Autodesk Inventor part; units mm, degrees
(part 3 of 4)
  line L749 (-36.8358, 2.1011) -> (-36.8212, 2.0626) construction
  line L750 (-36.8212, 2.0626) -> (-36.7965, 1.9968) construction
  line L751 (-36.7965, 1.9968) -> (-36.752, 1.9602) construction
  line L752 (-36.752, 1.9602) -> (-36.6802, 1.9558) construction
  line L753 (-36.6802, 1.9558) -> (-36.5155, 1.9456) construction
  line L754 (-36.5155, 1.9456) -> (-36.351, 1.9258) construction
  line L755 (-36.351, 1.9258) -> (-36.1863, 1.9252) construction
  line L756 (-36.1863, 1.9252) -> (-36.0465, 1.9246) construction
  line L757 (-36.0465, 1.9246) -> (-35.9064, 1.9438) construction
  line L758 (-35.9064, 1.9438) -> (-35.767, 1.9589) construction
  line L759 (-35.767, 1.9589) -> (-35.7495, 1.9609) construction
  line L760 (-35.7495, 1.9609) -> (-35.7233, 1.9899) construction
  line L761 (-35.7233, 1.9899) -> (-35.7209, 2.009) construction
  line L762 (-35.7209, 2.009) -> (-35.7008, 2.1678) construction
  line L763 (-35.7008, 2.1678) -> (-35.7931, 2.3069) construction
  line L764 (-35.7931, 2.3069) -> (-35.9501, 2.3398) construction
  line L765 (-35.9501, 2.3398) -> (-36.0921, 2.3695) construction
  line L766 (-36.0921, 2.3695) -> (-36.2371, 2.3846) construction
  line L767 (-36.2371, 2.3846) -> (-36.3665, 2.404) construction
  spline S6 degree 3 poles (-30.3554, -3.8594) (-30.3555, -3.8591) (-30.3549, -3.8478) (-30.3601, -3.8409) (-30.4995, -3.6571) (-30.6375, -3.472) (-30.7805, -3.291) (-30.8314, -3.2266) (-30.8561, -3.2345) (-30.8937, -3.311) (-30.9012, -3.3262) (-30.908, -3.3419) (-30.9132, -3.358) (-30.9647, -3.5173) (-31.0168, -3.6764) (-31.0665, -3.8362) (-31.0875, -3.9039) (-31.1033, -3.9732) (-31.1184, -4.0298) (-30.8621, -3.9726) (-30.6123, -3.9168) (-30.3554, -3.8594) knots 0 0 0 0 1 1 1 2 2 2 3 3 3 4 4 4 5 5 5 6 6 6 7 7 7 7
  line L768 (-30.3554, -3.8594) -> (-30.3555, -3.8591) construction
  line L769 (-30.3555, -3.8591) -> (-30.3549, -3.8478) construction
  line L770 (-30.3549, -3.8478) -> (-30.3601, -3.8409) construction
  line L771 (-30.3601, -3.8409) -> (-30.4995, -3.6571) construction
  line L772 (-30.4995, -3.6571) -> (-30.6375, -3.472) construction
  line L773 (-30.6375, -3.472) -> (-30.7805, -3.291) construction
  line L774 (-30.7805, -3.291) -> (-30.8314, -3.2266) construction
  line L775 (-30.8314, -3.2266) -> (-30.8561, -3.2345) construction
  line L776 (-30.8561, -3.2345) -> (-30.8937, -3.311) construction
  line L777 (-30.8937, -3.311) -> (-30.9012, -3.3262) construction
  line L778 (-30.9012, -3.3262) -> (-30.908, -3.3419) construction
  line L779 (-30.908, -3.3419) -> (-30.9132, -3.358) construction
  line L780 (-30.9132, -3.358) -> (-30.9647, -3.5173) construction
  line L781 (-30.9647, -3.5173) -> (-31.0168, -3.6764) construction
  line L782 (-31.0168, -3.6764) -> (-31.0665, -3.8362) construction
  line L783 (-31.0665, -3.8362) -> (-31.0875, -3.9039) construction
  line L784 (-31.0875, -3.9039) -> (-31.1033, -3.9732) construction
  line L785 (-31.1033, -3.9732) -> (-31.1184, -4.0298) construction
  line L786 (-31.1184, -4.0298) -> (-30.8621, -3.9726) construction
  line L787 (-30.8621, -3.9726) -> (-30.6123, -3.9168) construction
  line L788 (-30.6123, -3.9168) -> (-30.3554, -3.8594) construction
  spline S7 degree 3 poles (-13.1118, -0.4311) (-12.8875, -0.6685) (-12.6633, -0.8759) (-12.4133, -1.0565) (-12.4098, -0.9882) (-12.4138, -0.9278) (-12.4222, -0.868) (-12.4412, -0.7318) (-12.441, -0.5909) (-12.5232, -0.4699) (-12.578, -0.3894) (-12.6473, -0.3362) (-12.7483, -0.3537) (-12.8628, -0.3736) (-12.9758, -0.4017) (-13.1118, -0.4311) knots 0 0 0 0 1 1 1 2 2 2 3 3 3 4 4 4 5 5 5 5
  line L789 (-13.1118, -0.4311) -> (-12.8875, -0.6685) construction
  line L790 (-12.8875, -0.6685) -> (-12.6633, -0.8759) construction
  line L791 (-12.6633, -0.8759) -> (-12.4133, -1.0565) construction
  line L792 (-12.4133, -1.0565) -> (-12.4098, -0.9882) construction
  line L793 (-12.4098, -0.9882) -> (-12.4138, -0.9278) construction
  line L794 (-12.4138, -0.9278) -> (-12.4222, -0.868) construction
  line L795 (-12.4222, -0.868) -> (-12.4412, -0.7318) construction
  line L796 (-12.4412, -0.7318) -> (-12.441, -0.5909) construction
  line L797 (-12.441, -0.5909) -> (-12.5232, -0.4699) construction
  line L798 (-12.5232, -0.4699) -> (-12.578, -0.3894) construction
  line L799 (-12.578, -0.3894) -> (-12.6473, -0.3362) construction
  line L800 (-12.6473, -0.3362) -> (-12.7483, -0.3537) construction
  line L801 (-12.7483, -0.3537) -> (-12.8628, -0.3736) construction
  line L802 (-12.8628, -0.3736) -> (-12.9758, -0.4017) construction
  line L803 (-12.9758, -0.4017) -> (-13.1118, -0.4311) construction
  spline S8 degree 3 poles (-34.0058, 1.9385) (-33.8926, 1.9385) (-33.7872, 1.9385) (-33.6737, 1.9385) (-33.7306, 2.049) (-33.7865, 2.1577) (-33.8425, 2.2664) (-33.8504, 2.2656) (-33.8582, 2.2647) (-33.866, 2.2639) (-33.9126, 2.1556) (-33.9591, 2.0472) (-34.0058, 1.9385) knots 0 0 0 0 1 1 1 2 2 2 3 3 3 4 4 4 4
  line L804 (-34.0058, 1.9385) -> (-33.8926, 1.9385) construction
  line L805 (-33.8926, 1.9385) -> (-33.7872, 1.9385) construction
  line L806 (-33.7872, 1.9385) -> (-33.6737, 1.9385) construction
  line L807 (-33.6737, 1.9385) -> (-33.7306, 2.049) construction
  line L808 (-33.7306, 2.049) -> (-33.7865, 2.1577) construction
  line L809 (-33.7865, 2.1577) -> (-33.8425, 2.2664) construction
  line L810 (-33.8425, 2.2664) -> (-33.8504, 2.2656) construction
  line L811 (-33.8504, 2.2656) -> (-33.8582, 2.2647) construction
  line L812 (-33.8582, 2.2647) -> (-33.866, 2.2639) construction
  line L813 (-33.866, 2.2639) -> (-33.9126, 2.1556) construction
  line L814 (-33.9126, 2.1556) -> (-33.9591, 2.0472) construction
  line L815 (-33.9591, 2.0472) -> (-34.0058, 1.9385) construction
  spline S9 degree 3 poles (-35.895, -7.7567) (-36.1424, -7.7391) (-36.3938, -7.7434) (-36.6363, -7.6993) (-37.1289, -7.6097) (-37.4813, -7.3075) (-37.7375, -6.89) (-38.0544, -6.3737) (-38.2471, -5.8126) (-38.2894, -5.2073) (-38.3247, -4.7018) (-38.2191, -4.2311) (-37.867, -3.8444) (-37.5822, -3.5315) (-37.2197, -3.3455) (-36.8095, -3.2651) (-36.49, -3.2025) (-36.1657, -3.1617) (-35.842, -3.1253) (-35.4744, -3.0839) (-35.1055, -3.0519) (-34.7364, -3.0276) (-34.4733, -3.0103) (-34.2167, -3.0559) (-33.9756, -3.1681) (-33.9277, -3.1904) (-33.8818, -3.2213) (-33.8424, -3.2565) (-33.6743, -3.4066) (-33.677, -3.636) (-33.8413, -3.8231) (-33.992, -3.9948) (-34.192, -4.0671) (-34.4039, -4.126) (-34.668, -4.1992) (-34.9386, -4.1983) (-35.208, -4.2138) (-35.6243, -4.2377) (-36.0359, -4.2895) (-36.443, -4.3844) (-36.6934, -4.4428) (-36.8567, -4.5851) (-36.9532, -4.8174) (-37.174, -5.3491) (-37.1437, -5.8504) (-36.7631, -6.3017) (-36.4548, -6.6671) (-36.0468, -6.8064) (-35.5809, -6.7621) (-35.2569, -6.7312) (-34.9357, -6.6708) (-34.6137, -6.6206) (-34.4887, -6.6011) (-34.3656, -6.5701) (-34.2406, -6.5506) (-34.1678, -6.5392) (-34.1482, -6.5075) (-34.1621, -6.4365) (-34.2138, -6.1741) (-34.2642, -5.9114) (-34.3096, -5.6479) (-34.3525, -5.3991) (-34.3697, -5.1487) (-34.3, -4.9016) (-34.2818, -4.8372) (-34.2527, -4.7729) (-34.2153, -4.7175) (-34.1052, -4.5547) (-33.8905, -4.5308) (-33.7443, -4.6627) (-33.5657, -4.8237) (-33.4637, -5.0354) (-33.3765, -5.2522) (-33.2039, -5.6815) (-33.1123, -6.1314) (-33.0565, -6.5894) (-33.0471, -6.6667) (-33.0366, -6.7439) (-33.0232, -6.8206) (-32.966, -7.1464) (-33.1138, -7.3739) (-33.4413, -7.4318) (-33.8939, -7.5118) (-34.3486, -7.5799) (-34.8028, -7.6508) (-35.1642, -7.7073) (-35.5273, -7.7474) (-35.895, -7.7567) knots 0 0 0 0 1 1 1 2 2 2 3 3 3 4 4 4 5 5 5 6 6 6 7 7 7 8 8 8 9 9 9 10 10 10 11 11 11 12 12 12 13 13 13 14 14 14 15 15 15 16 16 16 17 17 17 18 18 18 19 19 19 20 20 20 21 21 21 22 22 22 23 23 23 24 24 24 25 25 25 26 26 26 27 27 27 28 28 28 29 29 29 29
  line L816 (-35.895, -7.7567) -> (-36.1424, -7.7391) construction
  line L817 (-36.1424, -7.7391) -> (-36.3938, -7.7434) construction
  line L818 (-36.3938, -7.7434) -> (-36.6363, -7.6993) construction
  line L819 (-36.6363, -7.6993) -> (-37.1289, -7.6097) construction
  line L820 (-37.1289, -7.6097) -> (-37.4813, -7.3075) construction
  line L821 (-37.4813, -7.3075) -> (-37.7375, -6.89) construction
  line L822 (-37.7375, -6.89) -> (-38.0544, -6.3737) construction
  line L823 (-38.0544, -6.3737) -> (-38.2471, -5.8126) construction
  line L824 (-38.2471, -5.8126) -> (-38.2894, -5.2073) construction
  line L825 (-38.2894, -5.2073) -> (-38.3247, -4.7018) construction
  line L826 (-38.3247, -4.7018) -> (-38.2191, -4.2311) construction
  line L827 (-38.2191, -4.2311) -> (-37.867, -3.8444) construction
  line L828 (-37.867, -3.8444) -> (-37.5822, -3.5315) construction
  line L829 (-37.5822, -3.5315) -> (-37.2197, -3.3455) construction
  line L830 (-37.2197, -3.3455) -> (-36.8095, -3.2651) construction
  line L831 (-36.8095, -3.2651) -> (-36.49, -3.2025) construction
  line L832 (-36.49, -3.2025) -> (-36.1657, -3.1617) construction
  line L833 (-36.1657, -3.1617) -> (-35.842, -3.1253) construction
  line L834 (-35.842, -3.1253) -> (-35.4744, -3.0839) construction
  line L835 (-35.4744, -3.0839) -> (-35.1055, -3.0519) construction
  line L836 (-35.1055, -3.0519) -> (-34.7364, -3.0276) construction
  line L837 (-34.7364, -3.0276) -> (-34.4733, -3.0103) construction
  line L838 (-34.4733, -3.0103) -> (-34.2167, -3.0559) construction
  line L839 (-34.2167, -3.0559) -> (-33.9756, -3.1681) construction
  line L840 (-33.9756, -3.1681) -> (-33.9277, -3.1904) construction
  line L841 (-33.9277, -3.1904) -> (-33.8818, -3.2213) construction
  line L842 (-33.8818, -3.2213) -> (-33.8424, -3.2565) construction
  line L843 (-33.8424, -3.2565) -> (-33.6743, -3.4066) construction
  line L844 (-33.6743, -3.4066) -> (-33.677, -3.636) construction
  line L845 (-33.677, -3.636) -> (-33.8413, -3.8231) construction
  line L846 (-33.8413, -3.8231) -> (-33.992, -3.9948) construction
  line L847 (-33.992, -3.9948) -> (-34.192, -4.0671) construction
  line L848 (-34.192, -4.0671) -> (-34.4039, -4.126) construction
  line L849 (-34.4039, -4.126) -> (-34.668, -4.1992) construction
  line L850 (-34.668, -4.1992) -> (-34.9386, -4.1983) construction
  line L851 (-34.9386, -4.1983) -> (-35.208, -4.2138) construction
  line L852 (-35.208, -4.2138) -> (-35.6243, -4.2377) construction
  line L853 (-35.6243, -4.2377) -> (-36.0359, -4.2895) construction
  line L854 (-36.0359, -4.2895) -> (-36.443, -4.3844) construction
  line L855 (-36.443, -4.3844) -> (-36.6934, -4.4428) construction
  line L856 (-36.6934, -4.4428) -> (-36.8567, -4.5851) construction
  line L857 (-36.8567, -4.5851) -> (-36.9532, -4.8174) construction
  line L858 (-36.9532, -4.8174) -> (-37.174, -5.3491) construction
  line L859 (-37.174, -5.3491) -> (-37.1437, -5.8504) construction
  line L860 (-37.1437, -5.8504) -> (-36.7631, -6.3017) construction
  line L861 (-36.7631, -6.3017) -> (-36.4548, -6.6671) construction
  line L862 (-36.4548, -6.6671) -> (-36.0468, -6.8064) construction
  line L863 (-36.0468, -6.8064) -> (-35.5809, -6.7621) construction
  line L864 (-35.5809, -6.7621) -> (-35.2569, -6.7312) construction
  line L865 (-35.2569, -6.7312) -> (-34.9357, -6.6708) construction
  line L866 (-34.9357, -6.6708) -> (-34.6137, -6.6206) construction
  line L867 (-34.6137, -6.6206) -> (-34.4887, -6.6011) construction
  line L868 (-34.4887, -6.6011) -> (-34.3656, -6.5701) construction
  line L869 (-34.3656, -6.5701) -> (-34.2406, -6.5506) construction
  line L870 (-34.2406, -6.5506) -> (-34.1678, -6.5392) construction
  line L871 (-34.1678, -6.5392) -> (-34.1482, -6.5075) construction
  line L872 (-34.1482, -6.5075) -> (-34.1621, -6.4365) construction
  line L873 (-34.1621, -6.4365) -> (-34.2138, -6.1741) construction
  line L874 (-34.2138, -6.1741) -> (-34.2642, -5.9114) construction
  line L875 (-34.2642, -5.9114) -> (-34.3096, -5.6479) construction
  line L876 (-34.3096, -5.6479) -> (-34.3525, -5.3991) construction
  line L877 (-34.3525, -5.3991) -> (-34.3697, -5.1487) construction
  line L878 (-34.3697, -5.1487) -> (-34.3, -4.9016) construction
  line L879 (-34.3, -4.9016) -> (-34.2818, -4.8372) construction
  line L880 (-34.2818, -4.8372) -> (-34.2527, -4.7729) construction
  line L881 (-34.2527, -4.7729) -> (-34.2153, -4.7175) construction
  line L882 (-34.2153, -4.7175) -> (-34.1052, -4.5547) construction
  line L883 (-34.1052, -4.5547) -> (-33.8905, -4.5308) construction
  line L884 (-33.8905, -4.5308) -> (-33.7443, -4.6627) construction
  line L885 (-33.7443, -4.6627) -> (-33.5657, -4.8237) construction
  line L886 (-33.5657, -4.8237) -> (-33.4637, -5.0354) construction
  line L887 (-33.4637, -5.0354) -> (-33.3765, -5.2522) construction
  line L888 (-33.3765, -5.2522) -> (-33.2039, -5.6815) construction
  line L889 (-33.2039, -5.6815) -> (-33.1123, -6.1314) construction
  line L890 (-33.1123, -6.1314) -> (-33.0565, -6.5894) construction
  line L891 (-33.0565, -6.5894) -> (-33.0471, -6.6667) construction
  line L892 (-33.0471, -6.6667) -> (-33.0366, -6.7439) construction
  line L893 (-33.0366, -6.7439) -> (-33.0232, -6.8206) construction
  line L894 (-33.0232, -6.8206) -> (-32.966, -7.1464) construction
  line L895 (-32.966, -7.1464) -> (-33.1138, -7.3739) construction
  line L896 (-33.1138, -7.3739) -> (-33.4413, -7.4318) construction
  line L897 (-33.4413, -7.4318) -> (-33.8939, -7.5118) construction
  line L898 (-33.8939, -7.5118) -> (-34.3486, -7.5799) construction
  line L899 (-34.3486, -7.5799) -> (-34.8028, -7.6508) construction
  line L900 (-34.8028, -7.6508) -> (-35.1642, -7.7073) construction
  line L901 (-35.1642, -7.7073) -> (-35.5273, -7.7474) construction
  line L902 (-35.5273, -7.7474) -> (-35.895, -7.7567) construction
  spline S10 degree 3 poles (-2.8177, 1.9833) (-2.5485, 1.9797) (-2.3514, 1.9723) (-2.1629, 1.9042) (-1.8782, 1.8014) (-1.772, 1.5571) (-1.8859, 1.2769) (-1.9292, 1.1704) (-2.006, 1.1171) (-2.1193, 1.1084) (-2.418, 1.0857) (-2.7172, 1.0676) (-3.015, 1.0358) (-3.3441, 1.0006) (-3.6708, 0.9468) (-3.9845, 0.8347) (-4.406, 0.6841) (-4.6415, 0.3807) (-4.6795, -0.0605) (-4.7351, -0.7055) (-4.5093, -1.2626) (-4.0911, -1.7412) (-3.855, -2.0113) (-3.5295, -2.1002) (-3.1828, -2.0681) (-2.844, -2.0367) (-2.5086, -1.9708) (-2.1711, -1.9238) (-1.9256, -1.8897) (-1.6799, -1.8454) (-1.4331, -1.8358) (-1.2234, -1.8277) (-1.0323, -1.9103) (-0.8865, -2.0717) (-0.7282, -2.2469) (-0.7355, -2.5112) (-0.9122, -2.6423) (-0.9791, -2.6918) (-1.0695, -2.7232) (-1.153, -2.7345) (-1.6234, -2.7985) (-2.0954, -2.8506) (-2.566, -2.9132) (-2.8935, -2.9568) (-3.2214, -2.9779) (-3.5497, -2.94) (-3.98, -2.8903) (-4.3813, -2.765) (-4.7095, -2.4618) (-5.0222, -2.173) (-5.2227, -1.8167) (-5.3497, -1.4157) (-5.5113, -0.9055) (-5.5908, -0.3833) (-5.5707, 0.1527) (-5.5426, 0.8984) (-5.1639, 1.3959) (-4.4856, 1.6781) (-4.1342, 1.8244) (-3.7605, 1.8795) (-3.3866, 1.9282) (-3.1743, 1.9558) (-2.9603, 1.9698) (-2.8177, 1.9833) knots 0 0 0 0 1 1 1 2 2 2 3 3 3 4 4 4 5 5 5 6 6 6 7 7 7 8 8 8 9 9 9 10 10 10 11 11 11 12 12 12 13 13 13 14 14 14 15 15 15 16 16 16 17 17 17 18 18 18 19 19 19 20 20 20 21 21 21 21
  line L903 (-2.8177, 1.9833) -> (-2.5485, 1.9797) construction
  line L904 (-2.5485, 1.9797) -> (-2.3514, 1.9723) construction
  line L905 (-2.3514, 1.9723) -> (-2.1629, 1.9042) construction
  line L906 (-2.1629, 1.9042) -> (-1.8782, 1.8014) construction
  line L907 (-1.8782, 1.8014) -> (-1.772, 1.5571) construction
  line L908 (-1.772, 1.5571) -> (-1.8859, 1.2769) construction
  line L909 (-1.8859, 1.2769) -> (-1.9292, 1.1704) construction
  line L910 (-1.9292, 1.1704) -> (-2.006, 1.1171) construction
  line L911 (-2.006, 1.1171) -> (-2.1193, 1.1084) construction
  line L912 (-2.1193, 1.1084) -> (-2.418, 1.0857) construction
  line L913 (-2.418, 1.0857) -> (-2.7172, 1.0676) construction
  line L914 (-2.7172, 1.0676) -> (-3.015, 1.0358) construction
  line L915 (-3.015, 1.0358) -> (-3.3441, 1.0006) construction
  line L916 (-3.3441, 1.0006) -> (-3.6708, 0.9468) construction
  line L917 (-3.6708, 0.9468) -> (-3.9845, 0.8347) construction
  line L918 (-3.9845, 0.8347) -> (-4.406, 0.6841) construction
  line L919 (-4.406, 0.6841) -> (-4.6415, 0.3807) construction
  line L920 (-4.6415, 0.3807) -> (-4.6795, -0.0605) construction
  line L921 (-4.6795, -0.0605) -> (-4.7351, -0.7055) construction
  line L922 (-4.7351, -0.7055) -> (-4.5093, -1.2626) construction
  line L923 (-4.5093, -1.2626) -> (-4.0911, -1.7412) construction
  line L924 (-4.0911, -1.7412) -> (-3.855, -2.0113) construction
  line L925 (-3.855, -2.0113) -> (-3.5295, -2.1002) construction
  line L926 (-3.5295, -2.1002) -> (-3.1828, -2.0681) construction
  line L927 (-3.1828, -2.0681) -> (-2.844, -2.0367) construction
  line L928 (-2.844, -2.0367) -> (-2.5086, -1.9708) construction
  line L929 (-2.5086, -1.9708) -> (-2.1711, -1.9238) construction
  line L930 (-2.1711, -1.9238) -> (-1.9256, -1.8897) construction
  line L931 (-1.9256, -1.8897) -> (-1.6799, -1.8454) construction
  line L932 (-1.6799, -1.8454) -> (-1.4331, -1.8358) construction
  line L933 (-1.4331, -1.8358) -> (-1.2234, -1.8277) construction
  line L934 (-1.2234, -1.8277) -> (-1.0323, -1.9103) construction
  line L935 (-1.0323, -1.9103) -> (-0.8865, -2.0717) construction
  line L936 (-0.8865, -2.0717) -> (-0.7282, -2.2469) construction
  line L937 (-0.7282, -2.2469) -> (-0.7355, -2.5112) construction
  line L938 (-0.7355, -2.5112) -> (-0.9122, -2.6423) construction
  line L939 (-0.9122, -2.6423) -> (-0.9791, -2.6918) construction
  line L940 (-0.9791, -2.6918) -> (-1.0695, -2.7232) construction
  line L941 (-1.0695, -2.7232) -> (-1.153, -2.7345) construction
  line L942 (-1.153, -2.7345) -> (-1.6234, -2.7985) construction
  line L943 (-1.6234, -2.7985) -> (-2.0954, -2.8506) construction
  line L944 (-2.0954, -2.8506) -> (-2.566, -2.9132) construction
  line L945 (-2.566, -2.9132) -> (-2.8935, -2.9568) construction
  line L946 (-2.8935, -2.9568) -> (-3.2214, -2.9779) construction
  line L947 (-3.2214, -2.9779) -> (-3.5497, -2.94) construction
  line L948 (-3.5497, -2.94) -> (-3.98, -2.8903) construction
  line L949 (-3.98, -2.8903) -> (-4.3813, -2.765) construction
  line L950 (-4.3813, -2.765) -> (-4.7095, -2.4618) construction
  line L951 (-4.7095, -2.4618) -> (-5.0222, -2.173) construction
  line L952 (-5.0222, -2.173) -> (-5.2227, -1.8167) construction
  line L953 (-5.2227, -1.8167) -> (-5.3497, -1.4157) construction
  line L954 (-5.3497, -1.4157) -> (-5.5113, -0.9055) construction
  line L955 (-5.5113, -0.9055) -> (-5.5908, -0.3833) construction
  line L956 (-5.5908, -0.3833) -> (-5.5707, 0.1527) construction
  line L957 (-5.5707, 0.1527) -> (-5.5426, 0.8984) construction
  line L958 (-5.5426, 0.8984) -> (-5.1639, 1.3959) construction
  line L959 (-5.1639, 1.3959) -> (-4.4856, 1.6781) construction
  line L960 (-4.4856, 1.6781) -> (-4.1342, 1.8244) construction
  line L961 (-4.1342, 1.8244) -> (-3.7605, 1.8795) construction
  line L962 (-3.7605, 1.8795) -> (-3.3866, 1.9282) construction
  line L963 (-3.3866, 1.9282) -> (-3.1743, 1.9558) construction
  line L964 (-3.1743, 1.9558) -> (-2.9603, 1.9698) construction
  line L965 (-2.9603, 1.9698) -> (-2.8177, 1.9833) construction
  spline S11 degree 3 poles (-10.8046, -2.6746) (-10.0622, -2.8966) (-9.3253, -3.1169) (-8.5835, -3.3387) (-8.5838, -3.3404) (-8.5839, -3.3524) (-8.5873, -3.3635) (-8.6584, -3.5989) (-8.473, -3.8294) (-8.2158, -3.8169) (-7.9978, -3.8063) (-7.7779, -3.7828) (-7.5647, -3.7375) (-7.3037, -3.6819) (-7.0583, -3.7064) (-6.8041, -3.7791) (-6.1028, -3.9797) (-5.3937, -4.1537) (-4.6943, -4.3607) (-3.9203, -4.5897) (-3.152, -4.8384) (-2.385, -5.0902) (-2.2024, -5.1502) (-2.0349, -5.2564) (-1.861, -5.3426) (-1.8401, -5.3529) (-1.823, -5.3711) (-1.8041, -5.3857) (-1.8031, -5.3941) (-1.8021, -5.4025) (-1.8011, -5.4109) (-1.8825, -5.4349) (-1.9626, -5.4714) (-2.0456, -5.4809) (-2.5658, -5.5397) (-3.0858, -5.6025) (-3.6074, -5.6442) (-4.0273, -5.6778) (-4.4493, -5.6851) (-4.8705, -5.7013) (-5.982, -5.7441) (-7.0916, -5.6664) (-8.2018, -5.6397) (-9.0279, -5.6198) (-9.8536, -5.5933) (-10.6798, -5.6092) (-11.5228, -5.6253) (-12.3452, -5.7674) (-13.1436, -6.0411) (-13.6663, -6.2202) (-14.1471, -6.484) (-14.6164, -6.7717) (-15.0953, -7.0654) (-15.5733, -7.361) (-16.0583, -7.6444) (-16.7344, -8.0394) (-17.4595, -8.3159) (-18.22, -8.4998) (-18.8161, -8.6439) (-19.4221, -8.7251) (-20.034, -8.7452) (-20.44, -8.7586) (-20.8485, -8.7604) (-21.2532, -8.7308) (-21.79, -8.6915) (-22.3167, -8.5793) (-22.8349, -8.4301) (-23.6204, -8.2039) (-24.3485, -7.8571) (-25.0219, -7.3949) (-25.376, -7.1519) (-25.7001, -6.8723) (-26.0081, -6.5737) (-26.0252, -6.5571) (-26.0389, -6.5371) (-26.067, -6.5032) (-25.9618, -6.4898) (-25.87, -6.4792) (-25.7786, -6.4663) (-24.9399, -6.3475) (-24.101, -6.2296) (-23.2803, -6.0122) (-23.0739, -5.9575) (-23.0018, -5.8099) (-23.0898, -5.6166) (-23.195, -5.3854) (-23.3911, -5.2725) (-23.6286, -5.2246) (-23.8956, -5.1707) (-24.1563, -5.2226) (-24.4153, -5.287) (-24.831, -5.3903) (-25.2463, -5.4967) (-25.6742, -5.5369) (-25.7949, -5.5483) (-25.9177, -5.551) (-26.0386, -5.5436) (-26.2543, -5.5304) (-26.4002, -5.4087) (-26.4629, -5.2082) (-26.5279, -4.9999) (-26.5735, -4.7852) (-26.6212, -4.5718) (-26.7294, -4.0879) (-26.8342, -3.6032) (-26.9392, -3.1186) (-26.9969, -2.8525) (-27.0474, -2.5847) (-27.1107, -2.3201) (-27.1473, -2.1672) (-27.1869, -2.012) (-27.3043, -1.8935) (-27.4144, -1.7824) (-27.5471, -1.7543) (-27.6939, -1.7885) (-27.8419, -1.823) (-27.9482, -1.9157) (-27.9718, -2.0652) (-27.9893, -2.1758) (-27.9801, -2.2942) (-27.9632, -2.4061) (-27.8782, -2.969) (-27.7858, -3.5307) (-27.6982, -4.0931) (-27.657, -4.3577) (-27.6204, -4.6229) (-27.5827, -4.888) (-27.5788, -4.9155) (-27.5822, -4.944) (-27.5822, -4.9924) (-27.6226, -4.9665) (-27.648, -4.9521) (-27.6712, -4.9349) (-27.9327, -4.7411) (-28.1812, -4.5258) (-28.4587, -4.3589) (-28.7294, -4.1961) (-28.9127, -3.9595) (-29.1131, -3.7318) (-29.5224, -3.2668) (-29.9506, -2.821) (-30.4548, -2.4553) (-30.5688, -2.3726) (-30.6949, -2.3159) (-30.8323, -2.2878) (-31.063, -2.2407) (-31.2437, -2.3292) (-31.3819, -2.5095) (-31.4631, -2.6156) (-31.5371, -2.7276) (-31.6079, -2.841) (-31.6405, -2.8931) (-31.6684, -2.9076) (-31.7305, -2.8878) (-32.5354, -2.6318) (-33.3526, -2.4216) (-34.1767, -2.2372) (-34.7108, -2.1178) (-35.2435, -1.9918) (-35.7788, -1.8784) (-36.3767, -1.7518) (-36.9677, -1.6025) (-37.5477, -1.4089) (-37.9807, -1.2643) (-38.4004, -1.092) (-38.7922, -0.8558) (-38.8114, -0.8442) (-38.8262, -0.8253) (-38.8431, -0.8098) (-38.8243, -0.7973) (-38.8072, -0.7804) (-38.7866, -0.773) (-38.4189, -0.6404) (-38.0343, -0.595) (-37.6486, -0.5569) (-36.8248, -0.4755) (-35.9986, -0.487) (-35.1725, -0.4937) (-34.8166, -0.4966) (-34.4607, -0.4912) (-34.1048, -0.4917) (-33.3492, -0.493) (-32.5935, -0.4951) (-31.8379, -0.4988) (-31.7805, -0.4991) (-31.7232, -0.5152) (-31.6656, -0.5218) (-31.6347, -0.5254) (-31.603, -0.5277) (-31.5721, -0.5251) (-31.4802, -0.5174) (-31.3887, -0.4997) (-31.2969, -0.499) (-30.7387, -0.4944) (-30.1801, -0.5069) (-29.6225, -0.4881) (-28.9059, -0.464) (-28.2067, -0.3296) (-27.5287, -0.0923) (-27.0196, 0.0859) (-26.5739, 0.3736) (-26.1481, 0.6983) (-25.7398, 1.0097) (-25.3363, 1.3289) (-24.9124, 1.618) (-24.3706, 1.9875) (-23.7885, 2.2873) (-23.1623, 2.4911) (-22.5798, 2.6806) (-21.9816, 2.7981) (-21.3726, 2.8668) (-20.8673, 2.9238) (-20.3614, 2.9449) (-19.8549, 2.906) (-19.5445, 2.8822) (-19.2333, 2.8493) (-18.9269, 2.7951) (-17.9224, 2.6173) (-16.9784, 2.2798) (-16.128, 1.7028) (-15.5463, 1.3081) (-15.0566, 0.8164) (-14.6061, 0.282) (-14.5529, 0.2189) (-14.4997, 0.1558) (-14.4527, 0.0999) (-14.4987, 0.0306) (-14.5536, -0.0307) (-14.5841, -0.1023) (-14.6622, -0.2857) (-14.5586, -0.4803) (-14.3617, -0.512) (-14.2353, -0.5324) (-14.1048, -0.5288) (-13.9761, -0.5314) (-13.9189, -0.5326) (-13.8769, -0.5484) (-13.8361, -0.5922) (-13.4224, -1.0367) (-12.9915, -1.4638) (-12.4777, -1.7932) (-12.3401, -1.8815) (-12.2917, -1.9874) (-12.271, -2.1401) (-12.1854, -2.772) (-12.0323, -3.3866) (-11.7608, -3.9671) (-11.6996, -4.0978) (-11.6301, -4.2262) (-11.5015, -4.3033) (-11.2778, -4.4375) (-10.9866, -4.3539) (-10.8435, -4.1189) (-10.7319, -3.9357) (-10.7136, -3.7324) (-10.7292, -3.526) (-10.75, -3.2493) (-10.7803, -2.9734) (-10.8063, -2.6971) (-10.8072, -2.6879) (-10.8049, -2.6785) (-10.8046, -2.6746) knots 0 0 0 0 1 1 1 2 2 2 3 3 3 4 4 4 5 5 5 6 6 6 7 7 7 8 8 8 9 9 9 10 10 10 11 11 11 12 12 12 13 13 13 14 14 14 15 15 15 16 16 16 17 17 17 18 18 18 19 19 19 20 20 20 21 21 21 22 22 22 23 23 23 24 24 24 25 25 25 26 26 26 27 27 27 28 28 28 29 29 29 30 30 30 31 31 31 32 32 32 33 33 33 34 34 34 35 35 35 36 36 36 37 37 37 38 38 38 39 39 39 40 40 40 41 41 41 42 42 42 43 43 43 44 44 44 45 45 45 46 46 46 47 47 47 48 48 48 49 49 49 50 50 50 51 51 51 52 52 52 53 53 53 54 54 54 55 55 55 56 56 56 57 57 57 58 58 58 59 59 59 60 60 60 61 61 61 62 62 62 63 63 63 64 64 64 65 65 65 66 66 66 67 67 67 68 68 68 69 69 69 70 70 70 71 71 71 72 72 72 73 73 73 74 74 74 75 75 75 76 76 76 77 77 77 78 78 78 79 79 79 80 80 80 81 81 81 82 82 82 83 83 83 84 84 84 85 85 85 86 86 86 87 87 87 87
  line L966 (-10.8046, -2.6746) -> (-10.0622, -2.8966) construction
  line L967 (-10.0622, -2.8966) -> (-9.3253, -3.1169) construction
  line L968 (-9.3253, -3.1169) -> (-8.5835, -3.3387) construction
  line L969 (-8.5835, -3.3387) -> (-8.5838, -3.3404) construction
  line L970 (-8.5838, -3.3404) -> (-8.5839, -3.3524) construction
  line L971 (-8.5839, -3.3524) -> (-8.5873, -3.3635) construction
  line L972 (-8.5873, -3.3635) -> (-8.6584, -3.5989) construction
  line L973 (-8.6584, -3.5989) -> (-8.473, -3.8294) construction
  line L974 (-8.473, -3.8294) -> (-8.2158, -3.8169) construction
  line L975 (-8.2158, -3.8169) -> (-7.9978, -3.8063) construction
  line L976 (-7.9978, -3.8063) -> (-7.7779, -3.7828) construction
  line L977 (-7.7779, -3.7828) -> (-7.5647, -3.7375) construction
  line L978 (-7.5647, -3.7375) -> (-7.3037, -3.6819) construction
  line L979 (-7.3037, -3.6819) -> (-7.0583, -3.7064) construction
  line L980 (-7.0583, -3.7064) -> (-6.8041, -3.7791) construction
  line L981 (-6.8041, -3.7791) -> (-6.1028, -3.9797) construction
  line L982 (-6.1028, -3.9797) -> (-5.3937, -4.1537) construction
  line L983 (-5.3937, -4.1537) -> (-4.6943, -4.3607) construction
  line L984 (-4.6943, -4.3607) -> (-3.9203, -4.5897) construction
  line L985 (-3.9203, -4.5897) -> (-3.152, -4.8384) construction
  line L986 (-3.152, -4.8384) -> (-2.385, -5.0902) construction
  line L987 (-2.385, -5.0902) -> (-2.2024, -5.1502) construction
  line L988 (-2.2024, -5.1502) -> (-2.0349, -5.2564) construction
  line L989 (-2.0349, -5.2564) -> (-1.861, -5.3426) construction
  line L990 (-1.861, -5.3426) -> (-1.8401, -5.3529) construction
  line L991 (-1.8401, -5.3529) -> (-1.823, -5.3711) construction
  line L992 (-1.823, -5.3711) -> (-1.8041, -5.3857) construction
  line L993 (-1.8041, -5.3857) -> (-1.8031, -5.3941) construction
  line L994 (-1.8031, -5.3941) -> (-1.8021, -5.4025) construction
  line L995 (-1.8021, -5.4025) -> (-1.8011, -5.4109) construction
  line L996 (-1.8011, -5.4109) -> (-1.8825, -5.4349) construction
  line L997 (-1.8825, -5.4349) -> (-1.9626, -5.4714) construction
  line L998 (-1.9626, -5.4714) -> (-2.0456, -5.4809) construction
  line L999 (-2.0456, -5.4809) -> (-2.5658, -5.5397) construction
  line L1000 (-2.5658, -5.5397) -> (-3.0858, -5.6025) construction
  line L1001 (-3.0858, -5.6025) -> (-3.6074, -5.6442) construction
  line L1002 (-3.6074, -5.6442) -> (-4.0273, -5.6778) construction
  line L1003 (-4.0273, -5.6778) -> (-4.4493, -5.6851) construction
  line L1004 (-4.4493, -5.6851) -> (-4.8705, -5.7013) construction
  line L1005 (-4.8705, -5.7013) -> (-5.982, -5.7441) construction
  line L1006 (-5.982, -5.7441) -> (-7.0916, -5.6664) construction
  line L1007 (-7.0916, -5.6664) -> (-8.2018, -5.6397) construction
  line L1008 (-8.2018, -5.6397) -> (-9.0279, -5.6198) construction
  line L1009 (-9.0279, -5.6198) -> (-9.8536, -5.5933) construction
  line L1010 (-9.8536, -5.5933) -> (-10.6798, -5.6092) construction
  line L1011 (-10.6798, -5.6092) -> (-11.5228, -5.6253) construction
  line L1012 (-11.5228, -5.6253) -> (-12.3452, -5.7674) construction
  line L1013 (-12.3452, -5.7674) -> (-13.1436, -6.0411) construction
  line L1014 (-13.1436, -6.0411) -> (-13.6663, -6.2202) construction
  line L1015 (-13.6663, -6.2202) -> (-14.1471, -6.484) construction
  line L1016 (-14.1471, -6.484) -> (-14.6164, -6.7717) construction
  line L1017 (-14.6164, -6.7717) -> (-15.0953, -7.0654) construction
  line L1018 (-15.0953, -7.0654) -> (-15.5733, -7.361) construction
  line L1019 (-15.5733, -7.361) -> (-16.0583, -7.6444) construction
  line L1020 (-16.0583, -7.6444) -> (-16.7344, -8.0394) construction
  line L1021 (-16.7344, -8.0394) -> (-17.4595, -8.3159) construction
  line L1022 (-17.4595, -8.3159) -> (-18.22, -8.4998) construction
  line L1023 (-18.22, -8.4998) -> (-18.8161, -8.6439) construction
  line L1024 (-18.8161, -8.6439) -> (-19.4221, -8.7251) construction
  line L1025 (-19.4221, -8.7251) -> (-20.034, -8.7452) construction
  line L1026 (-20.034, -8.7452) -> (-20.44, -8.7586) construction
  line L1027 (-20.44, -8.7586) -> (-20.8485, -8.7604) construction
  line L1028 (-20.8485, -8.7604) -> (-21.2532, -8.7308) construction
  line L1029 (-21.2532, -8.7308) -> (-21.79, -8.6915) construction
  line L1030 (-21.79, -8.6915) -> (-22.3167, -8.5793) construction
  line L1031 (-22.3167, -8.5793) -> (-22.8349, -8.4301) construction
  line L1032 (-22.8349, -8.4301) -> (-23.6204, -8.2039) construction
  line L1033 (-23.6204, -8.2039) -> (-24.3485, -7.8571) construction
  line L1034 (-24.3485, -7.8571) -> (-25.0219, -7.3949) construction
  line L1035 (-25.0219, -7.3949) -> (-25.376, -7.1519) construction
  line L1036 (-25.376, -7.1519) -> (-25.7001, -6.8723) construction
  line L1037 (-25.7001, -6.8723) -> (-26.0081, -6.5737) construction
  line L1038 (-26.0081, -6.5737) -> (-26.0252, -6.5571) construction
  line L1039 (-26.0252, -6.5571) -> (-26.0389, -6.5371) construction
  line L1040 (-26.0389, -6.5371) -> (-26.067, -6.5032) construction
  line L1041 (-26.067, -6.5032) -> (-25.9618, -6.4898) construction
  line L1042 (-25.9618, -6.4898) -> (-25.87, -6.4792) construction
  line L1043 (-25.87, -6.4792) -> (-25.7786, -6.4663) construction
  line L1044 (-25.7786, -6.4663) -> (-24.9399, -6.3475) construction
  line L1045 (-24.9399, -6.3475) -> (-24.101, -6.2296) construction
  line L1046 (-24.101, -6.2296) -> (-23.2803, -6.0122) construction
  line L1047 (-23.2803, -6.0122) -> (-23.0739, -5.9575) construction
  line L1048 (-23.0739, -5.9575) -> (-23.0018, -5.8099) construction
  line L1049 (-23.0018, -5.8099) -> (-23.0898, -5.6166) construction
  line L1050 (-23.0898, -5.6166) -> (-23.195, -5.3854) construction
  line L1051 (-23.195, -5.3854) -> (-23.3911, -5.2725) construction
  line L1052 (-23.3911, -5.2725) -> (-23.6286, -5.2246) construction
  line L1053 (-23.6286, -5.2246) -> (-23.8956, -5.1707) construction
  line L1054 (-23.8956, -5.1707) -> (-24.1563, -5.2226) construction
  line L1055 (-24.1563, -5.2226) -> (-24.4153, -5.287) construction
  line L1056 (-24.4153, -5.287) -> (-24.831, -5.3903) construction
  line L1057 (-24.831, -5.3903) -> (-25.2463, -5.4967) construction
  line L1058 (-25.2463, -5.4967) -> (-25.6742, -5.5369) construction
  line L1059 (-25.6742, -5.5369) -> (-25.7949, -5.5483) construction
  line L1060 (-25.7949, -5.5483) -> (-25.9177, -5.551) construction
  line L1061 (-25.9177, -5.551) -> (-26.0386, -5.5436) construction
  line L1062 (-26.0386, -5.5436) -> (-26.2543, -5.5304) construction
  line L1063 (-26.2543, -5.5304) -> (-26.4002, -5.4087) construction
  line L1064 (-26.4002, -5.4087) -> (-26.4629, -5.2082) construction
  line L1065 (-26.4629, -5.2082) -> (-26.5279, -4.9999) construction
  line L1066 (-26.5279, -4.9999) -> (-26.5735, -4.7852) construction
  line L1067 (-26.5735, -4.7852) -> (-26.6212, -4.5718) construction
  line L1068 (-26.6212, -4.5718) -> (-26.7294, -4.0879) construction
  line L1069 (-26.7294, -4.0879) -> (-26.8342, -3.6032) construction
  line L1070 (-26.8342, -3.6032) -> (-26.9392, -3.1186) construction
  line L1071 (-26.9392, -3.1186) -> (-26.9969, -2.8525) construction
  line L1072 (-26.9969, -2.8525) -> (-27.0474, -2.5847) construction
  line L1073 (-27.0474, -2.5847) -> (-27.1107, -2.3201) construction
  line L1074 (-27.1107, -2.3201) -> (-27.1473, -2.1672) construction
  line L1075 (-27.1473, -2.1672) -> (-27.1869, -2.012) construction
  line L1076 (-27.1869, -2.012) -> (-27.3043, -1.8935) construction
  line L1077 (-27.3043, -1.8935) -> (-27.4144, -1.7824) construction
  line L1078 (-27.4144, -1.7824) -> (-27.5471, -1.7543) construction
  line L1079 (-27.5471, -1.7543) -> (-27.6939, -1.7885) construction
  line L1080 (-27.6939, -1.7885) -> (-27.8419, -1.823) construction
  line L1081 (-27.8419, -1.823) -> (-27.9482, -1.9157) construction
  line L1082 (-27.9482, -1.9157) -> (-27.9718, -2.0652) construction
  line L1083 (-27.9718, -2.0652) -> (-27.9893, -2.1758) construction
  line L1084 (-27.9893, -2.1758) -> (-27.9801, -2.2942) construction
  line L1085 (-27.9801, -2.2942) -> (-27.9632, -2.4061) construction
  line L1086 (-27.9632, -2.4061) -> (-27.8782, -2.969) construction
  line L1087 (-27.8782, -2.969) -> (-27.7858, -3.5307) construction
  line L1088 (-27.7858, -3.5307) -> (-27.6982, -4.0931) construction
  line L1089 (-27.6982, -4.0931) -> (-27.657, -4.3577) construction
  line L1090 (-27.657, -4.3577) -> (-27.6204, -4.6229) construction
  line L1091 (-27.6204, -4.6229) -> (-27.5827, -4.888) construction
  line L1092 (-27.5827, -4.888) -> (-27.5788, -4.9155) construction
  line L1093 (-27.5788, -4.9155) -> (-27.5822, -4.944) construction
  line L1094 (-27.5822, -4.944) -> (-27.5822, -4.9924) construction
  line L1095 (-27.5822, -4.9924) -> (-27.6226, -4.9665) construction
  line L1096 (-27.6226, -4.9665) -> (-27.648, -4.9521) construction
  line L1097 (-27.648, -4.9521) -> (-27.6712, -4.9349) construction
  line L1098 (-27.6712, -4.9349) -> (-27.9327, -4.7411) construction
  line L1099 (-27.9327, -4.7411) -> (-28.1812, -4.5258) construction
  line L1100 (-28.1812, -4.5258) -> (-28.4587, -4.3589) construction
  line L1101 (-28.4587, -4.3589) -> (-28.7294, -4.1961) construction
  line L1102 (-28.7294, -4.1961) -> (-28.9127, -3.9595) construction
  line L1103 (-28.9127, -3.9595) -> (-29.1131, -3.7318) construction
  line L1104 (-29.1131, -3.7318) -> (-29.5224, -3.2668) construction
  line L1105 (-29.5224, -3.2668) -> (-29.9506, -2.821) construction
  line L1106 (-29.9506, -2.821) -> (-30.4548, -2.4553) construction
  line L1107 (-30.4548, -2.4553) -> (-30.5688, -2.3726) construction
  line L1108 (-30.5688, -2.3726) -> (-30.6949, -2.3159) construction
  line L1109 (-30.6949, -2.3159) -> (-30.8323, -2.2878) construction
  line L1110 (-30.8323, -2.2878) -> (-31.063, -2.2407) construction
  line L1111 (-31.063, -2.2407) -> (-31.2437, -2.3292) construction
  line L1112 (-31.2437, -2.3292) -> (-31.3819, -2.5095) construction
  line L1113 (-31.3819, -2.5095) -> (-31.4631, -2.6156) construction
  line L1114 (-31.4631, -2.6156) -> (-31.5371, -2.7276) construction
  line L1115 (-31.5371, -2.7276) -> (-31.6079, -2.841) construction
  line L1116 (-31.6079, -2.841) -> (-31.6405, -2.8931) construction
  line L1117 (-31.6405, -2.8931) -> (-31.6684, -2.9076) construction
  line L1118 (-31.6684, -2.9076) -> (-31.7305, -2.8878) construction
  line L1119 (-31.7305, -2.8878) -> (-32.5354, -2.6318) construction
  line L1120 (-32.5354, -2.6318) -> (-33.3526, -2.4216) construction
  line L1121 (-33.3526, -2.4216) -> (-34.1767, -2.2372) construction
  line L1122 (-34.1767, -2.2372) -> (-34.7108, -2.1178) construction
  line L1123 (-34.7108, -2.1178) -> (-35.2435, -1.9918) construction
  line L1124 (-35.2435, -1.9918) -> (-35.7788, -1.8784) construction
  line L1125 (-35.7788, -1.8784) -> (-36.3767, -1.7518) construction
  line L1126 (-36.3767, -1.7518) -> (-36.9677, -1.6025) construction
  line L1127 (-36.9677, -1.6025) -> (-37.5477, -1.4089) construction
  line L1128 (-37.5477, -1.4089) -> (-37.9807, -1.2643) construction
  line L1129 (-37.9807, -1.2643) -> (-38.4004, -1.092) construction
  line L1130 (-38.4004, -1.092) -> (-38.7922, -0.8558) construction
  line L1131 (-38.7922, -0.8558) -> (-38.8114, -0.8442) construction
  line L1132 (-38.8114, -0.8442) -> (-38.8262, -0.8253) construction
  line L1133 (-38.8262, -0.8253) -> (-38.8431, -0.8098) construction
  line L1134 (-38.8431, -0.8098) -> (-38.8243, -0.7973) construction
  line L1135 (-38.8243, -0.7973) -> (-38.8072, -0.7804) construction
  line L1136 (-38.8072, -0.7804) -> (-38.7866, -0.773) construction
  line L1137 (-38.7866, -0.773) -> (-38.4189, -0.6404) construction
  line L1138 (-38.4189, -0.6404) -> (-38.0343, -0.595) construction
  line L1139 (-38.0343, -0.595) -> (-37.6486, -0.5569) construction
  line L1140 (-37.6486, -0.5569) -> (-36.8248, -0.4755) construction
  line L1141 (-36.8248, -0.4755) -> (-35.9986, -0.487) construction
  line L1142 (-35.9986, -0.487) -> (-35.1725, -0.4937) construction
  line L1143 (-35.1725, -0.4937) -> (-34.8166, -0.4966) construction
  line L1144 (-34.8166, -0.4966) -> (-34.4607, -0.4912) construction
  line L1145 (-34.4607, -0.4912) -> (-34.1048, -0.4917) construction
  line L1146 (-34.1048, -0.4917) -> (-33.3492, -0.493) construction
  line L1147 (-33.3492, -0.493) -> (-32.5935, -0.4951) construction
  line L1148 (-32.5935, -0.4951) -> (-31.8379, -0.4988) construction
  line L1149 (-31.8379, -0.4988) -> (-31.7805, -0.4991) construction
  line L1150 (-31.7805, -0.4991) -> (-31.7232, -0.5152) construction
  line L1151 (-31.7232, -0.5152) -> (-31.6656, -0.5218) construction
  line L1152 (-31.6656, -0.5218) -> (-31.6347, -0.5254) construction
  line L1153 (-31.6347, -0.5254) -> (-31.603, -0.5277) construction
  line L1154 (-31.603, -0.5277) -> (-31.5721, -0.5251) construction
  line L1155 (-31.5721, -0.5251) -> (-31.4802, -0.5174) construction
  line L1156 (-31.4802, -0.5174) -> (-31.3887, -0.4997) construction
  line L1157 (-31.3887, -0.4997) -> (-31.2969, -0.499) construction
  line L1158 (-31.2969, -0.499) -> (-30.7387, -0.4944) construction
  line L1159 (-30.7387, -0.4944) -> (-30.1801, -0.5069) construction
  line L1160 (-30.1801, -0.5069) -> (-29.6225, -0.4881) construction
  line L1161 (-29.6225, -0.4881) -> (-28.9059, -0.464) construction
  line L1162 (-28.9059, -0.464) -> (-28.2067, -0.3296) construction
  line L1163 (-28.2067, -0.3296) -> (-27.5287, -0.0923) construction
  line L1164 (-27.5287, -0.0923) -> (-27.0196, 0.0859) construction
  line L1165 (-27.0196, 0.0859) -> (-26.5739, 0.3736) construction
  line L1166 (-26.5739, 0.3736) -> (-26.1481, 0.6983) construction
  line L1167 (-26.1481, 0.6983) -> (-25.7398, 1.0097) construction
  line L1168 (-25.7398, 1.0097) -> (-25.3363, 1.3289) construction
  line L1169 (-25.3363, 1.3289) -> (-24.9124, 1.618) construction
  line L1170 (-24.9124, 1.618) -> (-24.3706, 1.9875) construction
  line L1171 (-24.3706, 1.9875) -> (-23.7885, 2.2873) construction
  line L1172 (-23.7885, 2.2873) -> (-23.1623, 2.4911) construction
  line L1173 (-23.1623, 2.4911) -> (-22.5798, 2.6806) construction
  line L1174 (-22.5798, 2.6806) -> (-21.9816, 2.7981) construction
  line L1175 (-21.9816, 2.7981) -> (-21.3726, 2.8668) construction
  line L1176 (-21.3726, 2.8668) -> (-20.8673, 2.9238) construction
  line L1177 (-20.8673, 2.9238) -> (-20.3614, 2.9449) construction
  line L1178 (-20.3614, 2.9449) -> (-19.8549, 2.906) construction
  line L1179 (-19.8549, 2.906) -> (-19.5445, 2.8822) construction
  line L1180 (-19.5445, 2.8822) -> (-19.2333, 2.8493) construction
  line L1181 (-19.2333, 2.8493) -> (-18.9269, 2.7951) construction
  line L1182 (-18.9269, 2.7951) -> (-17.9224, 2.6173) construction
  line L1183 (-17.9224, 2.6173) -> (-16.9784, 2.2798) construction
  line L1184 (-16.9784, 2.2798) -> (-16.128, 1.7028) construction
  line L1185 (-16.128, 1.7028) -> (-15.5463, 1.3081) construction
  line L1186 (-15.5463, 1.3081) -> (-15.0566, 0.8164) construction
  line L1187 (-15.0566, 0.8164) -> (-14.6061, 0.282) construction
  line L1188 (-14.6061, 0.282) -> (-14.5529, 0.2189) construction
  line L1189 (-14.5529, 0.2189) -> (-14.4997, 0.1558) construction
  line L1190 (-14.4997, 0.1558) -> (-14.4527, 0.0999) construction
  line L1191 (-14.4527, 0.0999) -> (-14.4987, 0.0306) construction
  line L1192 (-14.4987, 0.0306) -> (-14.5536, -0.0307) construction
  line L1193 (-14.5536, -0.0307) -> (-14.5841, -0.1023) construction
  line L1194 (-14.5841, -0.1023) -> (-14.6622, -0.2857) construction
  line L1195 (-14.6622, -0.2857) -> (-14.5586, -0.4803) construction
  line L1196 (-14.5586, -0.4803) -> (-14.3617, -0.512) construction
  line L1197 (-14.3617, -0.512) -> (-14.2353, -0.5324) construction
  line L1198 (-14.2353, -0.5324) -> (-14.1048, -0.5288) construction
  line L1199 (-14.1048, -0.5288) -> (-13.9761, -0.5314) construction
  line L1200 (-13.9761, -0.5314) -> (-13.9189, -0.5326) construction
  line L1201 (-13.9189, -0.5326) -> (-13.8769, -0.5484) construction
  line L1202 (-13.8769, -0.5484) -> (-13.8361, -0.5922) construction
  line L1203 (-13.8361, -0.5922) -> (-13.4224, -1.0367) construction
  line L1204 (-13.4224, -1.0367) -> (-12.9915, -1.4638) construction
  line L1205 (-12.9915, -1.4638) -> (-12.4777, -1.7932) construction
  line L1206 (-12.4777, -1.7932) -> (-12.3401, -1.8815) construction
  line L1207 (-12.3401, -1.8815) -> (-12.2917, -1.9874) construction
  line L1208 (-12.2917, -1.9874) -> (-12.271, -2.1401) construction
  line L1209 (-12.271, -2.1401) -> (-12.1854, -2.772) construction
  line L1210 (-12.1854, -2.772) -> (-12.0323, -3.3866) construction
  line L1211 (-12.0323, -3.3866) -> (-11.7608, -3.9671) construction
  line L1212 (-11.7608, -3.9671) -> (-11.6996, -4.0978) construction
  line L1213 (-11.6996, -4.0978) -> (-11.6301, -4.2262) construction
  line L1214 (-11.6301, -4.2262) -> (-11.5015, -4.3033) construction
  line L1215 (-11.5015, -4.3033) -> (-11.2778, -4.4375) construction
  line L1216 (-11.2778, -4.4375) -> (-10.9866, -4.3539) construction
  line L1217 (-10.9866, -4.3539) -> (-10.8435, -4.1189) construction
  line L1218 (-10.8435, -4.1189) -> (-10.7319, -3.9357) construction
  line L1219 (-10.7319, -3.9357) -> (-10.7136, -3.7324) construction
  line L1220 (-10.7136, -3.7324) -> (-10.7292, -3.526) construction
  line L1221 (-10.7292, -3.526) -> (-10.75, -3.2493) construction
  line L1222 (-10.75, -3.2493) -> (-10.7803, -2.9734) construction
  line L1223 (-10.7803, -2.9734) -> (-10.8063, -2.6971) construction
  line L1224 (-10.8063, -2.6971) -> (-10.8072, -2.6879) construction
  line L1225 (-10.8072, -2.6879) -> (-10.8049, -2.6785) construction
  line L1226 (-10.8049, -2.6785) -> (-10.8046, -2.6746) construction
  spline S12 degree 3 poles (-22.9451, -5.2295) (-22.922, -5.3856) (-22.9076, -5.5437) (-22.8739, -5.6974) (-22.822, -5.9335) (-22.6144, -6.0184) (-22.4026, -5.8994) (-22.2207, -5.7972) (-22.096, -5.6385) (-21.9857, -5.4678) (-21.7813, -5.1515) (-21.6218, -4.8134) (-21.5075, -4.4542) (-21.4456, -4.2596) (-21.3508, -4.0829) (-21.2246, -3.9223) (-20.9998, -3.6362) (-20.612, -3.522) (-20.2668, -3.6352) (-19.9964, -3.7237) (-19.7992, -3.9064) (-19.6171, -4.1137) (-19.3663, -4.3991) (-19.1109, -4.6801) (-18.8006, -4.9046) (-18.6164, -5.0377) (-18.4268, -5.1605) (-18.2033, -5.2157) (-17.9236, -5.2848) (-17.7384, -5.1172) (-17.7696, -4.8335) (-17.8019, -4.5397) (-17.9125, -4.2741) (-18.055, -4.0201) (-18.3021, -3.5799) (-18.5873, -3.1648) (-18.8977, -2.7671) (-19.3209, -2.2247) (-19.771, -1.7065) (-20.302, -1.2657) (-20.4712, -1.1252) (-20.649, -0.9881) (-20.8417, -0.8844) (-21.1315, -0.7284) (-21.3936, -0.7965) (-21.5881, -1.0611) (-21.7129, -1.231) (-21.8333, -1.4082) (-21.9261, -1.5966) (-22.3628, -2.4829) (-22.6649, -3.4153) (-22.8444, -4.3866) (-22.8956, -4.6641) (-22.9442, -4.9431) (-22.9451, -5.2295) knots 0 0 0 0 1 1 1 2 2 2 3 3 3 4 4 4 5 5 5 6 6 6 7 7 7 8 8 8 9 9 9 10 10 10 11 11 11 12 12 12 13 13 13 14 14 14 15 15 15 16 16 16 17 17 17 18 18 18 18
  line L1227 (-22.9451, -5.2295) -> (-22.922, -5.3856) construction
  line L1228 (-22.922, -5.3856) -> (-22.9076, -5.5437) construction
  line L1229 (-22.9076, -5.5437) -> (-22.8739, -5.6974) construction
  line L1230 (-22.8739, -5.6974) -> (-22.822, -5.9335) construction
  line L1231 (-22.822, -5.9335) -> (-22.6144, -6.0184) construction
  line L1232 (-22.6144, -6.0184) -> (-22.4026, -5.8994) construction
  line L1233 (-22.4026, -5.8994) -> (-22.2207, -5.7972) construction
  line L1234 (-22.2207, -5.7972) -> (-22.096, -5.6385) construction
  line L1235 (-22.096, -5.6385) -> (-21.9857, -5.4678) construction
  line L1236 (-21.9857, -5.4678) -> (-21.7813, -5.1515) construction
  line L1237 (-21.7813, -5.1515) -> (-21.6218, -4.8134) construction
  line L1238 (-21.6218, -4.8134) -> (-21.5075, -4.4542) construction
  line L1239 (-21.5075, -4.4542) -> (-21.4456, -4.2596) construction
  line L1240 (-21.4456, -4.2596) -> (-21.3508, -4.0829) construction
  line L1241 (-21.3508, -4.0829) -> (-21.2246, -3.9223) construction
  line L1242 (-21.2246, -3.9223) -> (-20.9998, -3.6362) construction
  line L1243 (-20.9998, -3.6362) -> (-20.612, -3.522) construction
  line L1244 (-20.612, -3.522) -> (-20.2668, -3.6352) construction
  line L1245 (-20.2668, -3.6352) -> (-19.9964, -3.7237) construction
  line L1246 (-19.9964, -3.7237) -> (-19.7992, -3.9064) construction
  line L1247 (-19.7992, -3.9064) -> (-19.6171, -4.1137) construction
  line L1248 (-19.6171, -4.1137) -> (-19.3663, -4.3991) construction
  line L1249 (-19.3663, -4.3991) -> (-19.1109, -4.6801) construction
  line L1250 (-19.1109, -4.6801) -> (-18.8006, -4.9046) construction
  line L1251 (-18.8006, -4.9046) -> (-18.6164, -5.0377) construction
  line L1252 (-18.6164, -5.0377) -> (-18.4268, -5.1605) construction
  line L1253 (-18.4268, -5.1605) -> (-18.2033, -5.2157) construction
  line L1254 (-18.2033, -5.2157) -> (-17.9236, -5.2848) construction
  line L1255 (-17.9236, -5.2848) -> (-17.7384, -5.1172) construction
  line L1256 (-17.7384, -5.1172) -> (-17.7696, -4.8335) construction
  line L1257 (-17.7696, -4.8335) -> (-17.8019, -4.5397) construction
  line L1258 (-17.8019, -4.5397) -> (-17.9125, -4.2741) construction
  line L1259 (-17.9125, -4.2741) -> (-18.055, -4.0201) construction
  line L1260 (-18.055, -4.0201) -> (-18.3021, -3.5799) construction
  line L1261 (-18.3021, -3.5799) -> (-18.5873, -3.1648) construction
  line L1262 (-18.5873, -3.1648) -> (-18.8977, -2.7671) construction
  line L1263 (-18.8977, -2.7671) -> (-19.3209, -2.2247) construction
  line L1264 (-19.3209, -2.2247) -> (-19.771, -1.7065) construction
  line L1265 (-19.771, -1.7065) -> (-20.302, -1.2657) construction
  line L1266 (-20.302, -1.2657) -> (-20.4712, -1.1252) construction
  line L1267 (-20.4712, -1.1252) -> (-20.649, -0.9881) construction
  line L1268 (-20.649, -0.9881) -> (-20.8417, -0.8844) construction
  line L1269 (-20.8417, -0.8844) -> (-21.1315, -0.7284) construction
  line L1270 (-21.1315, -0.7284) -> (-21.3936, -0.7965) construction
  line L1271 (-21.3936, -0.7965) -> (-21.5881, -1.0611) construction
  line L1272 (-21.5881, -1.0611) -> (-21.7129, -1.231) construction
  line L1273 (-21.7129, -1.231) -> (-21.8333, -1.4082) construction
  line L1274 (-21.8333, -1.4082) -> (-21.9261, -1.5966) construction
  line L1275 (-21.9261, -1.5966) -> (-22.3628, -2.4829) construction
  line L1276 (-22.3628, -2.4829) -> (-22.6649, -3.4153) construction
  line L1277 (-22.6649, -3.4153) -> (-22.8444, -4.3866) construction
  line L1278 (-22.8444, -4.3866) -> (-22.8956, -4.6641) construction
  line L1279 (-22.8956, -4.6641) -> (-22.9442, -4.9431) construction
  line L1280 (-22.9442, -4.9431) -> (-22.9451, -5.2295) construction
  spline S13 degree 3 poles (-18.4071, -1.9562) (-18.4141, -1.9571) (-18.4211, -1.958) (-18.4281, -1.9589) (-18.3953, -2.224) (-18.3722, -2.4908) (-18.3273, -2.7539) (-18.2602, -3.146) (-18.1511, -3.5265) (-17.9502, -3.8747) (-17.7035, -4.3021) (-17.3591, -4.6088) (-16.8809, -4.76) (-16.5137, -4.8761) (-16.1388, -4.8972) (-15.7609, -4.8632) (-15.344, -4.8257) (-14.9284, -4.7723) (-14.5126, -4.7225) (-14.3097, -4.6982) (-14.1058, -4.6758) (-13.906, -4.6349) (-13.7036, -4.5936) (-13.5886, -4.433) (-13.6065, -4.2455) (-13.6174, -4.1315) (-13.6744, -4.0385) (-13.7549, -3.96) (-13.9237, -3.7955) (-14.1348, -3.7365) (-14.3597, -3.76) (-14.6956, -3.7951) (-15.0291, -3.8532) (-15.364, -3.8988) (-15.6048, -3.9316) (-15.8454, -3.9714) (-16.0874, -3.9874) (-16.4238, -4.0097) (-16.7238, -3.9011) (-16.9435, -3.6427) (-17.3408, -3.1754) (-17.5623, -2.6346) (-17.5206, -2.0131) (-17.4887, -1.5389) (-17.2384, -1.2172) (-16.7786, -1.0684) (-16.3846, -0.9409) (-15.9768, -0.89) (-15.5673, -0.8506) (-15.3662, -0.8312) (-15.164, -0.8225) (-14.9622, -0.8103) (-14.8743, -0.805) (-14.7969, -0.7758) (-14.7522, -0.6983) (-14.6073, -0.4469) (-14.6652, -0.192) (-14.9177, -0.0574) (-15.0775, 0.0278) (-15.2502, 0.0492) (-15.4261, 0.0563) (-15.7781, 0.0704) (-16.1265, 0.0344) (-16.473, -0.026) (-16.8039, -0.0836) (-17.133, -0.1458) (-17.439, -0.2941) (-17.8084, -0.4732) (-18.0982, -0.7312) (-18.265, -1.1138) (-18.3824, -1.3828) (-18.4168, -1.6658) (-18.4071, -1.9562) knots 0 0 0 0 1 1 1 2 2 2 3 3 3 4 4 4 5 5 5 6 6 6 7 7 7 8 8 8 9 9 9 10 10 10 11 11 11 12 12 12 13 13 13 14 14 14 15 15 15 16 16 16 17 17 17 18 18 18 19 19 19 20 20 20 21 21 21 22 22 22 23 23 23 24 24 24 24
  line L1281 (-18.4071, -1.9562) -> (-18.4141, -1.9571) construction
  line L1282 (-18.4141, -1.9571) -> (-18.4211, -1.958) construction
  line L1283 (-18.4211, -1.958) -> (-18.4281, -1.9589) construction
  line L1284 (-18.4281, -1.9589) -> (-18.3953, -2.224) construction
  line L1285 (-18.3953, -2.224) -> (-18.3722, -2.4908) construction
  line L1286 (-18.3722, -2.4908) -> (-18.3273, -2.7539) construction
  line L1287 (-18.3273, -2.7539) -> (-18.2602, -3.146) construction
  line L1288 (-18.2602, -3.146) -> (-18.1511, -3.5265) construction